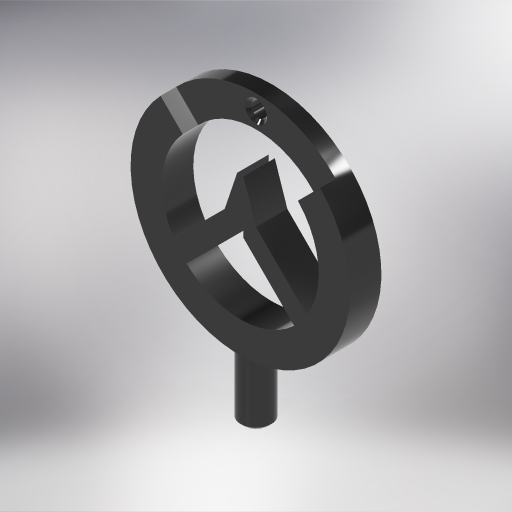
# Autodesk Inventor part: Black_Part1
Saved by Autodesk Inventor 2024 (Build 280153000, 153)
## iProperties
Created: 2023-10-30
Part Number: Black_Part1
Material: Generic
Document SubType Name: Modeling
Designer: SSAFY
Density: 1 g/cm^3
Appearance: Glossy - Black
Author: SSAFY
Autodesk Inventor part; units mm, degrees
ref_plane "YZ Plane" through (0, 0, 0) normal (1, 0, 0) x (0, 1, 0)
ref_plane "XY Plane" through (0, 0, 0) normal (0, 0, 1) x (1, 0, 0)
sketch "Sketch1" plane through (0, 0, 0) normal (0, 0, 1) x (1, 0, 0)
  circle A0 centre (0, 0) radius 25
  circle A1 centre (0, 0) radius 35
  line L0 (-17.6777, 17.6777) -> (-24.7487, 24.7487)
  line L1 (0, 35) -> (0, 0) construction
  line L2 (-24.0315, 25.4457) -> (-16.9564, 18.3706)
  line L3 (-1.1667, 34.9806) -> (-1.1667, 34.9972)
  line L4 (1.1667, 34.9806) -> (1.1667, 34.9972)
  line L5 (17.6777, 17.6777) -> (24.7487, 24.7487)
  line L6 (24.0315, 25.4457) -> (16.9564, 18.3706)
  line L7 (-25.4457, 24.0315) -> (-18.3706, 16.9564)
  line L8 (25.4457, 24.0315) -> (18.3706, 16.9564)
  line L9 (-1, 15) -> (1, 15)
  line L10 (1, 15) -> (1, 0)
  line L11 (1, 0) -> (-1, 0)
  line L12 (-1, 0) -> (-1, 15)
  line L13 (-1, 0) -> (1, 0)
  line L14 (1, 0) -> (1, -6)
  line L15 (1, -6) -> (-1, -6)
  line L16 (-1, -6) -> (-1, 0)
  line L17 (-1, -6) -> (-5, -6)
  line L18 (-5, -6) -> (-5, 3)
  line L19 (-5, 3) -> (-1, 3)
  line L20 (-1, 3) -> (-1, -6)
  line L21 (-5, 3) -> (-21.2192, -13.2192)
  line L22 (-5, -6) -> (-17.1706, -18.1706)
  line L23 (-5, 3) -> (-1, 15)
  line L24 (-5, -6) -> (-1, -2)
  line L25 (1, 0) -> (1, 15)
  line L26 (1, -6) -> (1, 0)
  line L27 (5, 3) -> (21.2192, -13.2192)
  line L28 (5, -6) -> (17.1706, -18.1706)
  line L29 (5, 3) -> (1, 15)
  line L30 (5, -6) -> (1, -2)
  point P0 (-20.5061, 21.9203)
  point P1 (-21.9203, 20.5061)
  point P2 (20.5061, 21.9203)
  point P3 (21.9203, 20.5061)
  point P4 (-1, -2)
  point P5 (1, 0)
  point P6 (1, -2)
  dimension "d0" = 50
  dimension "d1" = 10
  dimension "d2" = 45
  dimension "d3" = 1
  dimension "d5" = 2
  dimension "d6" = 15
  dimension "d7" = 6
  dimension "d8" = 2
  dimension "d9" = 4
  dimension "d11" = 45
  dimension "d12" = 45
  dimension "d13" = 3
  dimension "d14" = 45
  constraints: 62 end point, 8 symmetric about line, 6 parallel, 5 point on line, 3 horizontal, 3 perpendicular, 1 coincident, 1 midpoint, 1 vertical, 20 other
  measures "d2" angle of L1 L0
  measures "d3" distance between parallel lines of L2 L0
  measures "d5" distance of L9.start L9.end
  measures "d6" distance of L9.end L10.end
  measures "d7" distance of L13.end L14.end
  measures "d8" distance of L14.end L15.end
  measures "d9" distance of L15.end L17.end
  measures "d11" angle of L1 L21
  measures "d12" angle of L1 L22
  measures "d13" distance between parallel lines of L11 L19
  measures "d14" angle of L1 L24
extrude "Extrusion1" add sketch "Sketch1" along normal blind 10 contours A0 L8 A1 L7 | A0 L28 L30 L14 L10 L29 L27 | A0 L21 L18 L22 | L18 L19 L12 L16 L24 | L12 L19 L23
sketch "Sketch2" plane through (0, 0, 0) normal (0, 0, 1) x (1, 0, 0)
  point P0 (0, 0)
extrude "Extrusion2" add sketch "Sketch1" along normal blind 5 contours A0 L5 A1 L8 | A0 L6 A1 L5 | A0 L2 A1 L6 | A0 L0 A1 L2 | A1 L0 A0 L7
sketch "Sketch4" plane through (0, 0, 5) normal (0, 0, 1) x (1, 0, 0)
  arc A0 (18.3706, 16.9564) -> (-18.3706, 16.9564) centre (0, 0) ccw construction
  circle A1 centre (0, 30) radius 2.5
  point P0 (0, 25)
  dimension "d19" = 5
  dimension "d20" = 5
  constraints: 1 centre point, 1 point on circle
  measures "d19" diameter of A1
  measures "d20" distance of point (0, 25) A1.centre
extrude "Extrusion3" cut sketch "Sketch4" against normal through all
chamfer "Chamfer1" distance 1 angle 45 1 edges at (-2.5, 30, 5)
ref_plane "Work Plane1" through (0, -35, 0) normal (0, 1, 0) x (-1, 0, 0)
sketch "Sketch6" plane through (0, -35, 0) normal (0, 1, 0) x (-1, 0, 0)
  line L0 (3.5, 5) -> (-3.5, 5) construction
  circle A0 centre (0, 5) radius 4.9
  point P0 (0, 0)
  dimension "d27" = 9.8
  constraints: 1 centre point, 1 midpoint
  measures "d27" diameter of A0
extrude "Extrusion4" add sketch "Sketch6" along normal blind 5 and the other way blind 20
chamfer "Chamfer2" distance 1 angle 45 1 edges at (4.9, -55, 5)
body "Solid1"
